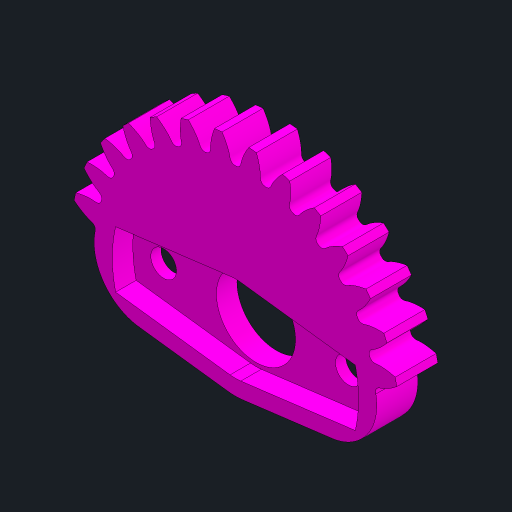
# Autodesk Inventor part: Servo Gear v3
Saved by Autodesk Inventor 2023.2 (Build 272271030, 271C)
## iProperties
Created: 2024-02-19
Part Number: Servo Gear v3
Material: Generic
Document SubType Name: Modeling
Designer: robpl
Density: 1 g/cm^3
Appearance: Magenta
Author: robpl
Autodesk Inventor part; units mm, degrees
ref_plane "YZ Plane" through (0, 0, 0) normal (1, 0, 0) x (0, 1, 0)
ref_plane "XZ Plane" through (0, 0, 0) normal (0, 1, 0) x (-1, 0, 0)
ref_plane "XY Plane" through (0, 0, 0) normal (0, 0, 1) x (1, 0, 0)
sketch "Sketch1" plane through (0, 0, 0) normal (0, 0, 1) x (1, 0, 0)
  spline S0 degree 3 poles (-1.3052, 15.9467) (-1.2453, 15.8516) (-1.1554, 15.709) (-1.0449, 15.5134) (-0.9655, 15.3647) (-0.8902, 15.2139) (-0.8193, 15.061) (-0.7533, 14.9059) (-0.6926, 14.7486) (-0.6381, 14.5891) (-0.5901, 14.4275) (-0.5589, 14.2906) (-0.5363, 14.1805) (-0.5125, 14.0995) (-0.4803, 14.0215) (-0.4383, 13.9482) (-0.3941, 13.8934) (-0.3542, 13.8537) (-0.3204, 13.8285) (-0.2858, 13.8043) (-0.2476, 13.7862) (-0.2089, 13.7695) (-0.1678, 13.7596) (-0.1265, 13.7512) (-0.0702, 13.7492) (0, 13.7505) (0.0702, 13.7492) (0.1265, 13.7512) (0.1678, 13.7596) (0.2089, 13.7695) (0.2476, 13.7862) (0.2858, 13.8043) (0.3204, 13.8285) (0.3542, 13.8537) (0.3941, 13.8934) (0.4383, 13.9482) (0.4803, 14.0215) (0.5125, 14.0995) (0.5363, 14.1805) (0.5589, 14.2906) (0.5901, 14.4275) (0.6381, 14.5891) (0.6926, 14.7486) (0.7533, 14.9059) (0.8193, 15.061) (0.8902, 15.2139) (0.9655, 15.3647) (1.0449, 15.5134) (1.1554, 15.709) (1.2453, 15.8516) (1.3052, 15.9467) knots 0 0 0 0 0.033702 0.050555 0.067407 0.084259 0.101111 0.117963 0.134815 0.151667 0.168518 0.185368 0.193792 0.202215 0.210638 0.219058 0.227476 0.231688 0.235901 0.240112 0.244326 0.248537 0.252749 0.256961 0.261174 0.2696 0.278026 0.282239 0.286451 0.290663 0.294874 0.299088 0.303299 0.307512 0.311724 0.320142 0.328562 0.336985 0.345408 0.353832 0.370682 0.387533 0.404385 0.421237 0.438089 0.454941 0.471793 0.488645 0.505498 0.5392 0.5392 0.5392 0.5392
  circle A0 centre (0, 0) radius 13.75 construction
  circle A1 centre (0, 0) radius 14.0954 construction
  circle A2 centre (0, 0) radius 15 construction
  circle A3 centre (0, 0) radius 16
  point P0 (-1.1285, 15.6597)
  point P1 (-1.0454, 15.513)
  point P2 (-0.9661, 15.3643)
  point P3 (-0.8909, 15.2135)
  point P4 (-0.8201, 15.0606)
  point P5 (-0.7542, 14.9055)
  point P6 (-0.6936, 14.7483)
  point P7 (-0.6392, 14.5888)
  point P8 (-0.5919, 14.4271)
  point P9 (-0.5535, 14.263)
  point P10 (-0.5352, 14.1808)
  point P11 (-0.5111, 14.1)
  point P12 (-0.4787, 14.0223)
  point P13 (-0.4365, 13.9494)
  point P14 (-0.3838, 13.8838)
  point P15 (-0.3535, 13.8545)
  point P16 (-0.3202, 13.8287)
  point P17 (-0.2852, 13.8053)
  point P18 (-0.2475, 13.7864)
  point P19 (-0.2085, 13.7706)
  point P20 (-0.1678, 13.7598)
  point P21 (-0.1263, 13.7524)
  point P22 (-0.0843, 13.75)
  point P23 (0, 13.75)
  point P24 (0.0843, 13.75)
  point P25 (0.1263, 13.7524)
  point P26 (0.1678, 13.7598)
  point P27 (0.2085, 13.7706)
  point P28 (0.2475, 13.7864)
  point P29 (0.2852, 13.8053)
  point P30 (0.3202, 13.8287)
  point P31 (0.3535, 13.8545)
  point P32 (0.3838, 13.8838)
  point P33 (0.4365, 13.9494)
  point P34 (0.4787, 14.0223)
  point P35 (0.5111, 14.1)
  point P36 (0.5352, 14.1808)
  point P37 (0.5535, 14.263)
  point P38 (0.5919, 14.4271)
  point P39 (0.6392, 14.5888)
  point P40 (0.6936, 14.7483)
  point P41 (0.7542, 14.9055)
  point P42 (0.8201, 15.0606)
  point P43 (0.8909, 15.2135)
  point P44 (0.9661, 15.3643)
  point P45 (1.0454, 15.513)
  point P46 (1.1285, 15.6597)
  constraints: 4 centre point, 2 point on circle, 103 other
extrude "Extrusion1" add sketch "Sketch1" against normal blind 4
extrude "Extrusion2" cut sketch "Sketch1" against normal through all contours A3 S0 picked at (-0.1198, 15.1654)
pattern_circular "Circular Pattern1" count 30 over 360 about axis through (0, 0, 0) along (0, 0, -1) of "Extrusion2"
sketch "Sketch2" plane through (0, 0, 0) normal (0, 0, 1) x (1, 0, 0)
  line L0 (-16, 0) -> (16, 0)
  arc A0 (-16.25, 1.9843) -> (-16.25, -1.9843) centre (-16, 0) ccw
  arc A1 (16.25, -1.9843) -> (16.25, 1.9843) centre (16, 0) ccw
  line L1 (0.5, 3.9686) -> (16.25, 1.9843)
  line L2 (16.25, -1.9843) -> (0.5, -3.9686)
  line L3 (-0.5, -3.9686) -> (-16.25, -1.9843)
  line L4 (-16.25, 1.9843) -> (-0.5, 3.9686)
  arc A2 (-0.5, -3.9686) -> (0.5, -3.9686) centre (0, 0) ccw
  arc A3 (0.5, 3.9686) -> (-0.5, 3.9686) centre (0, 0) ccw
  line L5 (16.275, 2.1827) -> (0.525, 4.1671)
  arc A4 (0.525, 4.1671) -> (-0.525, 4.1671) centre (0, 0) ccw
  line L6 (-0.525, 4.1671) -> (-16.275, 2.1827)
  arc A5 (-16.275, 2.1827) -> (-16.275, -2.1827) centre (-16, 0) ccw
  line L7 (-16.275, -2.1827) -> (-0.525, -4.1671)
  arc A6 (-0.525, -4.1671) -> (0.525, -4.1671) centre (0, 0) ccw
  line L8 (0.525, -4.1671) -> (16.275, -2.1827)
  arc A7 (16.275, -2.1827) -> (16.275, 2.1827) centre (16, 0) ccw
  circle A8 centre (0, 0) radius 12
  point P0 (11.6778, 2.7619)
  point P1 (-11.6778, 2.7619)
  point P2 (-11.6778, -2.7619)
  point P3 (11.6778, -2.7619)
  dimension "d8" = 32
  dimension "d9" = 4
  dimension "d10" = 4
  dimension "d11" = 4
  dimension "d12" = 0.2
  dimension "d13" = 24
  constraints: 18 end point, 16 point on circle, 9 centre point, 5 coincident, 5 tangent, 4 parallel, 1 horizontal, 1 midpoint, 7 other
  measures "d8" distance of L0.start L0.end
  measures "d9" diameter of A0
  measures "d10" diameter of A1
  measures "d11" radius of A2
  measures "d12" distance between parallel lines of L1 L5
  measures "d13" diameter of A8
extrude "Extrusion3" cut sketch "Sketch2" against normal blind 2 contours A8 L4 A3 L1 L0 | L0 A8 L2 A2 L3 | A8 L6 A4 L5 L1 A3 L4 | L3 A2 L2 A8 L8 A6 L7
sketch "Sketch3" plane through (0, 0, -2) normal (0, 0, 1) x (1, 0, 0)
  circle A0 centre (0, 0) radius 4.2
  line L0 (0.525, 4.1671) -> (11.6778, 2.7619) projected
  circle A1 centre (0, 0) radius 3.85
  dimension "d31" = 7.7
  constraints: 2 coincident, 1 centre point, 3 other
  measures "d31" diameter of A1
extrude "Extrusion4" cut sketch "Sketch3" against normal through all contours A1
sketch "Sketch4" plane through (0, 0, -4) normal (0, 0, -1) x (-1, 0, 0)
  point P0 (0, 0)
  point P1 (-9, 0)
  point P2 (9, 0)
  dimension "d18" = 18
  dimension "d19" = 9
  constraints: 2 horizontal alignment
  measures "d18" distance of point (-9, 0) point (9, 0)
  measures "d19" distance of point (0, 0) point (-9, 0)
hole "Hole1" at (9, 0, -4) at (-9, 0, -4) direction (0, 0, 1) diameter 2.5 end through all counterbore diameter 6 counterbore depth 1
sketch "Sketch6" plane through (0, 0, 0) normal (0, 0, 1) x (1, 0, 0)
  arc A0 (0.525, 4.1671) -> (-0.525, 4.1671) centre (0, 0) ccw projected
  line L0 (0.525, 4.1671) -> (11.6778, 2.7619) projected
  arc A1 (11.6778, -2.7619) -> (11.6778, 2.7619) centre (0, 0) ccw projected
  line L1 (11.6778, -2.7619) -> (0.525, -4.1671) projected
  line L2 (-0.525, -4.1671) -> (-11.6778, -2.7619) projected
  arc A2 (-11.6778, 2.7619) -> (-11.6778, -2.7619) centre (0, 0) ccw projected
  line L3 (-11.6778, 2.7619) -> (-0.525, 4.1671) projected
  arc A3 (-4.5922, 15.3268) -> (-5.2937, 15.0989) centre (0, 0) ccw projected
  arc A4 (-7.6784, 14.0371) -> (-8.3173, 13.6683) centre (0, 0) ccw projected
  arc A5 (-10.4291, 12.134) -> (-10.9773, 11.6404) centre (0, 0) ccw projected
  arc A6 (-12.724, 9.7005) -> (-13.1576, 9.1037) centre (0, 0) ccw projected
  arc A7 (-14.4628, 6.843) -> (-14.7629, 6.1691) centre (0, 0) ccw projected
  arc A8 (-15.5695, 3.6865) -> (-15.7229, 2.9649) centre (0, 0) ccw projected
  spline S0 degree 3 poles (-15.7229, 2.9649) (-15.6346, 2.8954) (-15.5022, 2.7911) (-15.3192, 2.6607) (-15.1796, 2.5662) (-15.0375, 2.4756) (-14.8928, 2.3892) (-14.7455, 2.3073) (-14.5954, 2.2305) (-14.4425, 2.1596) (-14.2868, 2.095) (-14.1538, 2.0496) (-14.0467, 2.0157) (-13.9687, 1.9835) (-13.8945, 1.9433) (-13.8259, 1.8939) (-13.7761, 1.8442) (-13.7408, 1.8003) (-13.7193, 1.7641) (-13.6988, 1.7271) (-13.6848, 1.6873) (-13.6722, 1.647) (-13.6667, 1.6052) (-13.6627, 1.5632) (-13.6666, 1.507) (-13.6752, 1.4373) (-13.6812, 1.3674) (-13.6891, 1.3116) (-13.7017, 1.2714) (-13.7159, 1.2316) (-13.7366, 1.1948) (-13.7586, 1.1587) (-13.7862, 1.1269) (-13.8149, 1.0959) (-13.8584, 1.0603) (-13.9176, 1.022) (-13.9949, 0.988) (-14.0759, 0.9641) (-14.1589, 0.9489) (-14.2707, 0.9379) (-14.4102, 0.9212) (-14.5759, 0.8904) (-14.7402, 0.8528) (-14.903, 0.8089) (-15.0641, 0.7594) (-15.2236, 0.705) (-15.3815, 0.6459) (-15.5376, 0.5825) (-15.7438, 0.493) (-15.895, 0.4185) (-15.9957, 0.3688) knots 0 0 0 0 0.062504 0.093759 0.125013 0.156267 0.187521 0.218774 0.250028 0.281281 0.312533 0.343783 0.359406 0.375028 0.39065 0.406265 0.421876 0.429689 0.437502 0.445312 0.453126 0.460936 0.468749 0.47656 0.484373 0.5 0.515627 0.52344 0.531251 0.539064 0.546874 0.554688 0.562498 0.570311 0.578124 0.593735 0.60935 0.624972 0.640594 0.656217 0.687467 0.718719 0.749972 0.781226 0.812479 0.843733 0.874987 0.906241 0.937496 1 1 1 1 projected
  arc A9 (-15.9957, 0.3688) -> (-15.9957, -0.3688) centre (0, 0) ccw projected
  spline S1 degree 3 poles (-15.9957, -0.3688) (-15.895, -0.4185) (-15.7438, -0.493) (-15.5376, -0.5825) (-15.3815, -0.6459) (-15.2236, -0.705) (-15.0641, -0.7594) (-14.903, -0.8089) (-14.7402, -0.8528) (-14.5759, -0.8904) (-14.4102, -0.9212) (-14.2707, -0.9379) (-14.1589, -0.9489) (-14.0759, -0.9641) (-13.9949, -0.988) (-13.9176, -1.022) (-13.8584, -1.0603) (-13.8149, -1.0959) (-13.7862, -1.1269) (-13.7586, -1.1587) (-13.7366, -1.1948) (-13.7159, -1.2316) (-13.7017, -1.2714) (-13.6891, -1.3116) (-13.6812, -1.3674) (-13.6752, -1.4373) (-13.6666, -1.507) (-13.6627, -1.5632) (-13.6667, -1.6052) (-13.6722, -1.647) (-13.6848, -1.6873) (-13.6988, -1.7271) (-13.7193, -1.7641) (-13.7408, -1.8003) (-13.7761, -1.8442) (-13.8259, -1.8939) (-13.8945, -1.9433) (-13.9687, -1.9835) (-14.0467, -2.0157) (-14.1538, -2.0496) (-14.2868, -2.095) (-14.4425, -2.1596) (-14.5954, -2.2305) (-14.7455, -2.3073) (-14.8928, -2.3892) (-15.0375, -2.4756) (-15.1796, -2.5662) (-15.3192, -2.6607) (-15.5022, -2.7911) (-15.6346, -2.8954) (-15.7229, -2.9649) knots 0 0 0 0 0.062504 0.093759 0.125013 0.156267 0.187521 0.218774 0.250028 0.281281 0.312533 0.343783 0.359406 0.375028 0.39065 0.406265 0.421876 0.429689 0.437502 0.445312 0.453126 0.460936 0.468749 0.47656 0.484373 0.5 0.515627 0.52344 0.531251 0.539064 0.546874 0.554688 0.562498 0.570311 0.578124 0.593735 0.60935 0.624972 0.640594 0.656217 0.687467 0.718719 0.749972 0.781226 0.812479 0.843733 0.874987 0.906241 0.937496 1 1 1 1 projected
  arc A10 (-15.7229, -2.9649) -> (-15.5695, -3.6865) centre (0, 0) ccw projected
  spline S2 degree 3 poles (-15.5695, -3.6865) (-15.4606, -3.7141) (-15.2972, -3.7555) (-15.077, -3.8002) (-14.911, -3.8298) (-14.7444, -3.8547) (-14.577, -3.8749) (-14.4091, -3.8897) (-14.2408, -3.8989) (-14.0723, -3.9014) (-13.9037, -3.8971) (-13.7638, -3.8845) (-13.6522, -3.8719) (-13.5678, -3.8696) (-13.4837, -3.8761) (-13.401, -3.8933) (-13.3352, -3.9185) (-13.2851, -3.9442) (-13.2507, -3.9685) (-13.217, -3.994) (-13.188, -4.0247) (-13.1601, -4.0564) (-13.138, -4.0923) (-13.1173, -4.1291) (-13.098, -4.182) (-13.0775, -4.2491) (-13.0546, -4.3155) (-13.0391, -4.3696) (-13.0343, -4.4116) (-13.031, -4.4537) (-13.035, -4.4957) (-13.0404, -4.5375) (-13.0527, -4.5779) (-13.0662, -4.6179) (-13.0916, -4.6681) (-13.13, -4.7271) (-13.1869, -4.7897) (-13.2511, -4.8444) (-13.3207, -4.8921) (-13.4184, -4.9476) (-13.539, -5.0196) (-13.6779, -5.1152) (-13.8128, -5.2163) (-13.9435, -5.3226) (-14.0706, -5.4333) (-14.1942, -5.548) (-14.3144, -5.6662) (-14.4312, -5.7876) (-14.5832, -5.9532) (-14.691, -6.0827) (-14.7629, -6.1691) knots 0 0 0 0 0.062504 0.093759 0.125013 0.156267 0.187521 0.218774 0.250028 0.281281 0.312533 0.343783 0.359406 0.375028 0.39065 0.406265 0.421876 0.429689 0.437502 0.445312 0.453126 0.460936 0.468749 0.47656 0.484373 0.5 0.515627 0.52344 0.531251 0.539064 0.546874 0.554688 0.562498 0.570311 0.578124 0.593735 0.60935 0.624972 0.640594 0.656217 0.687467 0.718719 0.749972 0.781226 0.812479 0.843733 0.874987 0.906241 0.937496 1 1 1 1 projected
  arc A11 (-14.7629, -6.1691) -> (-14.4628, -6.843) centre (0, 0) ccw projected
  spline S3 degree 3 poles (-14.4628, -6.843) (-14.3505, -6.8474) (-14.1821, -6.8539) (-13.9574, -6.8518) (-13.789, -6.8462) (-13.6207, -6.836) (-13.4528, -6.8209) (-13.2855, -6.8005) (-13.119, -6.7745) (-12.9536, -6.742) (-12.7897, -6.7027) (-12.6554, -6.6613) (-12.5488, -6.6258) (-12.4668, -6.6059) (-12.3832, -6.5948) (-12.2987, -6.5945) (-12.2291, -6.6054) (-12.1748, -6.6202) (-12.136, -6.6368) (-12.0978, -6.6547) (-12.063, -6.6787) (-12.0292, -6.7039) (-12.0001, -6.7344) (-11.9721, -6.7661) (-11.9423, -6.8138) (-11.9083, -6.8753) (-11.8721, -6.9354) (-11.8457, -6.9851) (-11.8322, -7.0251) (-11.8203, -7.0656) (-11.8154, -7.1076) (-11.812, -7.1496) (-11.8156, -7.1917) (-11.8206, -7.2336) (-11.8349, -7.288) (-11.8603, -7.3537) (-11.9029, -7.4267) (-11.9543, -7.4936) (-12.0125, -7.5547) (-12.0965, -7.6293) (-12.1995, -7.7248) (-12.3155, -7.8472) (-12.4264, -7.9741) (-12.5322, -8.1053) (-12.6335, -8.2401) (-12.7305, -8.3779) (-12.8235, -8.5185) (-12.9125, -8.6616) (-13.0267, -8.8551) (-13.1053, -9.0042) (-13.1576, -9.1037) knots 0 0 0 0 0.062504 0.093759 0.125013 0.156267 0.187521 0.218774 0.250028 0.281281 0.312533 0.343783 0.359406 0.375028 0.39065 0.406265 0.421876 0.429689 0.437502 0.445312 0.453126 0.460936 0.468749 0.47656 0.484373 0.5 0.515627 0.52344 0.531251 0.539064 0.546874 0.554688 0.562498 0.570311 0.578124 0.593735 0.60935 0.624972 0.640594 0.656217 0.687467 0.718719 0.749972 0.781226 0.812479 0.843733 0.874987 0.906241 0.937496 1 1 1 1 projected
  arc A12 (-13.1576, -9.1037) -> (-12.724, -9.7005) centre (0, 0) ccw projected
  spline S4 degree 3 poles (-12.724, -9.7005) (-12.6133, -9.6814) (-12.4472, -9.6528) (-12.2278, -9.604) (-12.0642, -9.5635) (-11.9018, -9.5185) (-11.7407, -9.4689) (-11.5813, -9.4142) (-11.4238, -9.354) (-11.2688, -9.2878) (-11.1166, -9.2153) (-10.9939, -9.1469) (-10.897, -9.09) (-10.8209, -9.0536) (-10.7414, -9.0253) (-10.6588, -9.0074) (-10.5885, -9.0036) (-10.5323, -9.0068) (-10.491, -9.015) (-10.4498, -9.0245) (-10.4109, -9.0408) (-10.3725, -9.0584) (-10.3377, -9.0822) (-10.3038, -9.1074) (-10.2646, -9.1479) (-10.2186, -9.2009) (-10.1707, -9.2522) (-10.1345, -9.2953) (-10.1131, -9.3317) (-10.093, -9.3688) (-10.0795, -9.4088) (-10.0674, -9.4493) (-10.0622, -9.4912) (-10.0584, -9.5332) (-10.0611, -9.5894) (-10.0722, -9.6589) (-10.0986, -9.7392) (-10.1351, -9.8153) (-10.1793, -9.8872) (-10.246, -9.9776) (-10.3269, -10.0924) (-10.4149, -10.2362) (-10.4969, -10.3835) (-10.5732, -10.5338) (-10.6442, -10.6866) (-10.7105, -10.8416) (-10.7722, -10.9985) (-10.8295, -11.1569) (-10.901, -11.37) (-10.9468, -11.5322) (-10.9773, -11.6404) knots 0 0 0 0 0.062504 0.093759 0.125013 0.156267 0.187521 0.218774 0.250028 0.281281 0.312533 0.343783 0.359406 0.375028 0.39065 0.406265 0.421876 0.429689 0.437502 0.445312 0.453126 0.460936 0.468749 0.47656 0.484373 0.5 0.515627 0.52344 0.531251 0.539064 0.546874 0.554688 0.562498 0.570311 0.578124 0.593735 0.60935 0.624972 0.640594 0.656217 0.687467 0.718719 0.749972 0.781226 0.812479 0.843733 0.874987 0.906241 0.937496 1 1 1 1 projected
  arc A13 (-10.9773, -11.6404) -> (-10.4291, -12.134) centre (0, 0) ccw projected
  spline S5 degree 3 poles (-10.4291, -12.134) (-10.3248, -12.0923) (-10.1683, -12.0298) (-9.9638, -11.9364) (-9.8122, -11.8628) (-9.6627, -11.785) (-9.5155, -11.703) (-9.3709, -11.6163) (-9.2294, -11.5248) (-9.0915, -11.4278) (-8.9577, -11.3252) (-8.8519, -11.2328) (-8.769, -11.157) (-8.7021, -11.1055) (-8.6302, -11.0613) (-8.5532, -11.0267) (-8.4852, -11.0083) (-8.4295, -10.9997) (-8.3874, -10.9992) (-8.3452, -10.9999) (-8.3037, -11.0077) (-8.2625, -11.017) (-8.2235, -11.0331) (-8.1851, -11.0506) (-8.1384, -11.0821) (-8.0824, -11.1244) (-8.0248, -11.1646) (-7.9805, -11.1993) (-7.9519, -11.2304) (-7.9245, -11.2625) (-7.903, -11.2988) (-7.8828, -11.3359) (-7.869, -11.3758) (-7.8565, -11.4161) (-7.8475, -11.4716) (-7.8439, -11.542) (-7.8531, -11.626) (-7.8729, -11.708) (-7.9012, -11.7875) (-7.9476, -11.8898) (-8.0029, -12.019) (-8.0591, -12.1779) (-8.1087, -12.339) (-8.152, -12.5019) (-8.1897, -12.6662) (-8.2223, -12.8315) (-8.2501, -12.9978) (-8.2732, -13.1647) (-8.2988, -13.388) (-8.3099, -13.5562) (-8.3173, -13.6683) knots 0 0 0 0 0.062504 0.093759 0.125013 0.156267 0.187521 0.218774 0.250028 0.281281 0.312533 0.343783 0.359406 0.375028 0.39065 0.406265 0.421876 0.429689 0.437502 0.445312 0.453126 0.460936 0.468749 0.47656 0.484373 0.5 0.515627 0.52344 0.531251 0.539064 0.546874 0.554688 0.562498 0.570311 0.578124 0.593735 0.60935 0.624972 0.640594 0.656217 0.687467 0.718719 0.749972 0.781226 0.812479 0.843733 0.874987 0.906241 0.937496 1 1 1 1 projected
  arc A14 (-8.3173, -13.6683) -> (-7.6784, -14.0371) centre (0, 0) ccw projected
  spline S6 degree 3 poles (-7.6784, -14.0371) (-7.585, -13.9747) (-7.4449, -13.881) (-7.2644, -13.7472) (-7.1314, -13.6437) (-7.0013, -13.5365) (-6.8744, -13.4256) (-6.751, -13.3108) (-6.6315, -13.1918) (-6.5169, -13.0683) (-6.4073, -12.9402) (-6.3231, -12.8277) (-6.2577, -12.7364) (-6.203, -12.6721) (-6.1419, -12.614) (-6.0737, -12.564) (-6.011, -12.5319) (-5.9584, -12.512) (-5.9172, -12.5027) (-5.8758, -12.4946) (-5.8336, -12.4936) (-5.7914, -12.4941) (-5.7498, -12.5017) (-5.7087, -12.5109) (-5.6564, -12.532) (-5.5928, -12.5617) (-5.5282, -12.5891) (-5.4776, -12.6138) (-5.4432, -12.6383) (-5.4097, -12.664) (-5.3811, -12.6951) (-5.3537, -12.7271) (-5.3319, -12.7633) (-5.3113, -12.8001) (-5.2909, -12.8525) (-5.2728, -12.9206) (-5.2643, -13.0047) (-5.2666, -13.089) (-5.2777, -13.1727) (-5.3019, -13.2824) (-5.3291, -13.4202) (-5.351, -13.5874) (-5.3661, -13.7553) (-5.3746, -13.9236) (-5.3773, -14.0921) (-5.3748, -14.2607) (-5.3674, -14.429) (-5.3553, -14.5971) (-5.334, -14.8209) (-5.3098, -14.9877) (-5.2937, -15.0989) knots 0 0 0 0 0.062504 0.093759 0.125013 0.156267 0.187521 0.218774 0.250028 0.281281 0.312533 0.343783 0.359406 0.375028 0.39065 0.406265 0.421876 0.429689 0.437502 0.445312 0.453126 0.460936 0.468749 0.47656 0.484373 0.5 0.515627 0.52344 0.531251 0.539064 0.546874 0.554688 0.562498 0.570311 0.578124 0.593735 0.60935 0.624972 0.640594 0.656217 0.687467 0.718719 0.749972 0.781226 0.812479 0.843733 0.874987 0.906241 0.937496 1 1 1 1 projected
  arc A15 (-5.2937, -15.0989) -> (-4.5922, -15.3268) centre (0, 0) ccw projected
  spline S7 degree 3 poles (-4.5922, -15.3268) (-4.5138, -15.2463) (-4.3962, -15.1255) (-4.2474, -14.9571) (-4.1389, -14.8282) (-4.0339, -14.6963) (-3.9328, -14.5615) (-3.836, -14.4235) (-3.7439, -14.2823) (-3.6574, -14.1377) (-3.5769, -13.9895) (-3.5179, -13.8621) (-3.4729, -13.7591) (-3.4328, -13.6849) (-3.3851, -13.6153) (-3.3288, -13.5522) (-3.2741, -13.5078) (-3.2268, -13.4774) (-3.1885, -13.4597) (-3.1496, -13.4432) (-3.1085, -13.4335) (-3.0671, -13.4252) (-3.0249, -13.424) (-2.9827, -13.4244) (-2.9273, -13.4342) (-2.8589, -13.45) (-2.79, -13.4634) (-2.7353, -13.477) (-2.6966, -13.4938) (-2.6585, -13.512) (-2.6241, -13.5365) (-2.5906, -13.5621) (-2.5617, -13.5929) (-2.5339, -13.6246) (-2.5031, -13.6717) (-2.4712, -13.7345) (-2.4454, -13.815) (-2.4301, -13.898) (-2.4237, -13.9821) (-2.4245, -14.0945) (-2.4224, -14.2349) (-2.4091, -14.403) (-2.3889, -14.5703) (-2.3622, -14.7368) (-2.3299, -14.9022) (-2.2924, -15.0665) (-2.2501, -15.2297) (-2.2034, -15.3916) (-2.136, -15.606) (-2.0777, -15.7641) (-2.0388, -15.8696) knots 0 0 0 0 0.062504 0.093759 0.125013 0.156267 0.187521 0.218774 0.250028 0.281281 0.312533 0.343783 0.359406 0.375028 0.39065 0.406265 0.421876 0.429689 0.437502 0.445312 0.453126 0.460936 0.468749 0.47656 0.484373 0.5 0.515627 0.52344 0.531251 0.539064 0.546874 0.554688 0.562498 0.570311 0.578124 0.593735 0.60935 0.624972 0.640594 0.656217 0.687467 0.718719 0.749972 0.781226 0.812479 0.843733 0.874987 0.906241 0.937496 1 1 1 1 projected
  arc A16 (-2.0388, -15.8696) -> (-1.3052, -15.9467) centre (0, 0) ccw projected
  spline S8 degree 3 poles (-1.3052, -15.9467) (-1.2453, -15.8516) (-1.1554, -15.709) (-1.0449, -15.5134) (-0.9655, -15.3647) (-0.8902, -15.2139) (-0.8193, -15.061) (-0.7533, -14.9059) (-0.6926, -14.7486) (-0.6381, -14.5891) (-0.5901, -14.4275) (-0.5589, -14.2906) (-0.5363, -14.1805) (-0.5125, -14.0995) (-0.4803, -14.0215) (-0.4383, -13.9482) (-0.3941, -13.8934) (-0.3542, -13.8537) (-0.3204, -13.8285) (-0.2858, -13.8043) (-0.2476, -13.7862) (-0.2089, -13.7695) (-0.1678, -13.7596) (-0.1265, -13.7512) (-0.0702, -13.7492) (0, -13.7505) (0.0702, -13.7492) (0.1265, -13.7512) (0.1678, -13.7596) (0.2089, -13.7695) (0.2476, -13.7862) (0.2858, -13.8043) (0.3204, -13.8285) (0.3542, -13.8537) (0.3941, -13.8934) (0.4383, -13.9482) (0.4803, -14.0215) (0.5125, -14.0995) (0.5363, -14.1805) (0.5589, -14.2906) (0.5901, -14.4275) (0.6381, -14.5891) (0.6926, -14.7486) (0.7533, -14.9059) (0.8193, -15.061) (0.8902, -15.2139) (0.9655, -15.3647) (1.0449, -15.5134) (1.1554, -15.709) (1.2453, -15.8516) (1.3052, -15.9467) knots 0 0 0 0 0.062504 0.093759 0.125013 0.156267 0.187521 0.218774 0.250028 0.281281 0.312533 0.343783 0.359406 0.375028 0.39065 0.406265 0.421876 0.429689 0.437502 0.445312 0.453126 0.460936 0.468749 0.47656 0.484373 0.5 0.515627 0.52344 0.531251 0.539064 0.546874 0.554688 0.562498 0.570311 0.578124 0.593735 0.60935 0.624972 0.640594 0.656217 0.687467 0.718719 0.749972 0.781226 0.812479 0.843733 0.874987 0.906241 0.937496 1 1 1 1 projected
  arc A17 (1.3052, -15.9467) -> (2.0388, -15.8696) centre (0, 0) ccw projected
  spline S9 degree 3 poles (2.0388, -15.8696) (2.0777, -15.7641) (2.136, -15.606) (2.2034, -15.3916) (2.2501, -15.2297) (2.2924, -15.0665) (2.3299, -14.9022) (2.3622, -14.7368) (2.3889, -14.5703) (2.4091, -14.403) (2.4224, -14.2349) (2.4245, -14.0945) (2.4237, -13.9821) (2.4301, -13.898) (2.4454, -13.815) (2.4712, -13.7345) (2.5031, -13.6717) (2.5339, -13.6246) (2.5617, -13.5929) (2.5906, -13.5621) (2.6241, -13.5365) (2.6585, -13.512) (2.6966, -13.4938) (2.7353, -13.477) (2.79, -13.4634) (2.8589, -13.45) (2.9273, -13.4342) (2.9827, -13.4244) (3.0249, -13.424) (3.0671, -13.4252) (3.1085, -13.4335) (3.1496, -13.4432) (3.1885, -13.4597) (3.2268, -13.4774) (3.2741, -13.5078) (3.3288, -13.5522) (3.3851, -13.6153) (3.4328, -13.6849) (3.4729, -13.7591) (3.5179, -13.8621) (3.5769, -13.9895) (3.6574, -14.1377) (3.7439, -14.2823) (3.836, -14.4235) (3.9328, -14.5615) (4.0339, -14.6963) (4.1389, -14.8282) (4.2474, -14.9571) (4.3962, -15.1255) (4.5138, -15.2463) (4.5922, -15.3268) knots 0 0 0 0 0.062504 0.093759 0.125013 0.156267 0.187521 0.218774 0.250028 0.281281 0.312533 0.343783 0.359406 0.375028 0.39065 0.406265 0.421876 0.429689 0.437502 0.445312 0.453126 0.460936 0.468749 0.47656 0.484373 0.5 0.515627 0.52344 0.531251 0.539064 0.546874 0.554688 0.562498 0.570311 0.578124 0.593735 0.60935 0.624972 0.640594 0.656217 0.687467 0.718719 0.749972 0.781226 0.812479 0.843733 0.874987 0.906241 0.937496 1 1 1 1 projected
  arc A18 (4.5922, -15.3268) -> (5.2937, -15.0989) centre (0, 0) ccw projected
  spline S10 degree 3 poles (5.2937, -15.0989) (5.3098, -14.9877) (5.334, -14.8209) (5.3553, -14.5971) (5.3674, -14.429) (5.3748, -14.2607) (5.3773, -14.0921) (5.3746, -13.9236) (5.3661, -13.7553) (5.351, -13.5874) (5.3291, -13.4202) (5.3019, -13.2824) (5.2777, -13.1727) (5.2666, -13.089) (5.2643, -13.0047) (5.2728, -12.9206) (5.2909, -12.8525) (5.3113, -12.8001) (5.3319, -12.7633) (5.3537, -12.7271) (5.3811, -12.6951) (5.4097, -12.664) (5.4432, -12.6383) (5.4776, -12.6138) (5.5282, -12.5891) (5.5928, -12.5617) (5.6564, -12.532) (5.7087, -12.5109) (5.7498, -12.5017) (5.7914, -12.4941) (5.8336, -12.4936) (5.8758, -12.4946) (5.9172, -12.5027) (5.9584, -12.512) (6.011, -12.5319) (6.0737, -12.564) (6.1419, -12.614) (6.203, -12.6721) (6.2577, -12.7364) (6.3231, -12.8277) (6.4073, -12.9402) (6.5169, -13.0683) (6.6315, -13.1918) (6.751, -13.3108) (6.8744, -13.4256) (7.0013, -13.5365) (7.1314, -13.6437) (7.2644, -13.7472) (7.4449, -13.881) (7.585, -13.9747) (7.6784, -14.0371) knots 0 0 0 0 0.062504 0.093759 0.125013 0.156267 0.187521 0.218774 0.250028 0.281281 0.312533 0.343783 0.359406 0.375028 0.39065 0.406265 0.421876 0.429689 0.437502 0.445312 0.453126 0.460936 0.468749 0.47656 0.484373 0.5 0.515627 0.52344 0.531251 0.539064 0.546874 0.554688 0.562498 0.570311 0.578124 0.593735 0.60935 0.624972 0.640594 0.656217 0.687467 0.718719 0.749972 0.781226 0.812479 0.843733 0.874987 0.906241 0.937496 1 1 1 1 projected
  arc A19 (7.6784, -14.0371) -> (8.3173, -13.6683) centre (0, 0) ccw projected
  spline S11 degree 3 poles (8.3173, -13.6683) (8.3099, -13.5562) (8.2988, -13.388) (8.2732, -13.1647) (8.2501, -12.9978) (8.2223, -12.8315) (8.1897, -12.6662) (8.152, -12.5019) (8.1087, -12.339) (8.0591, -12.1779) (8.0029, -12.019) (7.9476, -11.8898) (7.9012, -11.7875) (7.8729, -11.708) (7.8531, -11.626) (7.8439, -11.542) (7.8475, -11.4716) (7.8565, -11.4161) (7.869, -11.3758) (7.8828, -11.3359) (7.903, -11.2988) (7.9245, -11.2625) (7.9519, -11.2304) (7.9805, -11.1993) (8.0248, -11.1646) (8.0824, -11.1244) (8.1384, -11.0821) (8.1851, -11.0506) (8.2235, -11.0331) (8.2625, -11.017) (8.3037, -11.0077) (8.3452, -10.9999) (8.3874, -10.9992) (8.4295, -10.9997) (8.4852, -11.0083) (8.5532, -11.0267) (8.6302, -11.0613) (8.7021, -11.1055) (8.769, -11.157) (8.8519, -11.2328) (8.9577, -11.3252) (9.0915, -11.4278) (9.2294, -11.5248) (9.3709, -11.6163) (9.5155, -11.703) (9.6627, -11.785) (9.8122, -11.8628) (9.9638, -11.9364) (10.1683, -12.0298) (10.3248, -12.0923) (10.4291, -12.134) knots 0 0 0 0 0.062504 0.093759 0.125013 0.156267 0.187521 0.218774 0.250028 0.281281 0.312533 0.343783 0.359406 0.375028 0.39065 0.406265 0.421876 0.429689 0.437502 0.445312 0.453126 0.460936 0.468749 0.47656 0.484373 0.5 0.515627 0.52344 0.531251 0.539064 0.546874 0.554688 0.562498 0.570311 0.578124 0.593735 0.60935 0.624972 0.640594 0.656217 0.687467 0.718719 0.749972 0.781226 0.812479 0.843733 0.874987 0.906241 0.937496 1 1 1 1 projected
  arc A20 (10.4291, -12.134) -> (10.9773, -11.6404) centre (0, 0) ccw projected
  spline S12 degree 3 poles (10.9773, -11.6404) (10.9468, -11.5322) (10.901, -11.37) (10.8295, -11.1569) (10.7722, -10.9985) (10.7105, -10.8416) (10.6442, -10.6866) (10.5732, -10.5338) (10.4969, -10.3835) (10.4149, -10.2362) (10.3269, -10.0924) (10.246, -9.9776) (10.1793, -9.8872) (10.1351, -9.8153) (10.0986, -9.7392) (10.0722, -9.6589) (10.0611, -9.5894) (10.0584, -9.5332) (10.0622, -9.4912) (10.0674, -9.4493) (10.0795, -9.4088) (10.093, -9.3688) (10.1131, -9.3317) (10.1345, -9.2953) (10.1707, -9.2522) (10.2186, -9.2009) (10.2646, -9.1479) (10.3038, -9.1074) (10.3377, -9.0822) (10.3725, -9.0584) (10.4109, -9.0408) (10.4498, -9.0245) (10.491, -9.015) (10.5323, -9.0068) (10.5885, -9.0036) (10.6588, -9.0074) (10.7414, -9.0253) (10.8209, -9.0536) (10.897, -9.09) (10.9939, -9.1469) (11.1166, -9.2153) (11.2688, -9.2878) (11.4238, -9.354) (11.5813, -9.4142) (11.7407, -9.4689) (11.9018, -9.5185) (12.0642, -9.5635) (12.2278, -9.604) (12.4472, -9.6528) (12.6133, -9.6814) (12.724, -9.7005) knots 0 0 0 0 0.062504 0.093759 0.125013 0.156267 0.187521 0.218774 0.250028 0.281281 0.312533 0.343783 0.359406 0.375028 0.39065 0.406265 0.421876 0.429689 0.437502 0.445312 0.453126 0.460936 0.468749 0.47656 0.484373 0.5 0.515627 0.52344 0.531251 0.539064 0.546874 0.554688 0.562498 0.570311 0.578124 0.593735 0.60935 0.624972 0.640594 0.656217 0.687467 0.718719 0.749972 0.781226 0.812479 0.843733 0.874987 0.906241 0.937496 1 1 1 1 projected
  arc A21 (12.724, -9.7005) -> (13.1576, -9.1037) centre (0, 0) ccw projected
  spline S13 degree 3 poles (13.1576, -9.1037) (13.1053, -9.0042) (13.0267, -8.8551) (12.9125, -8.6616) (12.8235, -8.5185) (12.7305, -8.3779) (12.6335, -8.2401) (12.5322, -8.1053) (12.4264, -7.9741) (12.3155, -7.8472) (12.1995, -7.7248) (12.0965, -7.6293) (12.0125, -7.5547) (11.9543, -7.4936) (11.9029, -7.4267) (11.8603, -7.3537) (11.8349, -7.288) (11.8206, -7.2336) (11.8156, -7.1917) (11.812, -7.1496) (11.8154, -7.1076) (11.8203, -7.0656) (11.8322, -7.0251) (11.8457, -6.9851) (11.8721, -6.9354) (11.9083, -6.8753) (11.9423, -6.8138) (11.9721, -6.7661) (12.0001, -6.7344) (12.0292, -6.7039) (12.063, -6.6787) (12.0978, -6.6547) (12.136, -6.6368) (12.1748, -6.6202) (12.2291, -6.6054) (12.2987, -6.5945) (12.3832, -6.5948) (12.4668, -6.6059) (12.5488, -6.6258) (12.6554, -6.6613) (12.7897, -6.7027) (12.9536, -6.742) (13.119, -6.7745) (13.2855, -6.8005) (13.4528, -6.8209) (13.6207, -6.836) (13.789, -6.8462) (13.9574, -6.8518) (14.1821, -6.8539) (14.3505, -6.8474) (14.4628, -6.843) knots 0 0 0 0 0.062504 0.093759 0.125013 0.156267 0.187521 0.218774 0.250028 0.281281 0.312533 0.343783 0.359406 0.375028 0.39065 0.406265 0.421876 0.429689 0.437502 0.445312 0.453126 0.460936 0.468749 0.47656 0.484373 0.5 0.515627 0.52344 0.531251 0.539064 0.546874 0.554688 0.562498 0.570311 0.578124 0.593735 0.60935 0.624972 0.640594 0.656217 0.687467 0.718719 0.749972 0.781226 0.812479 0.843733 0.874987 0.906241 0.937496 1 1 1 1 projected
  arc A22 (14.4628, -6.843) -> (14.7629, -6.1691) centre (0, 0) ccw projected
  spline S14 degree 3 poles (14.7629, -6.1691) (14.691, -6.0827) (14.5832, -5.9532) (14.4312, -5.7876) (14.3144, -5.6662) (14.1942, -5.548) (14.0706, -5.4333) (13.9435, -5.3226) (13.8128, -5.2163) (13.6779, -5.1152) (13.539, -5.0196) (13.4184, -4.9476) (13.3207, -4.8921) (13.2511, -4.8444) (13.1869, -4.7897) (13.13, -4.7271) (13.0916, -4.6681) (13.0662, -4.6179) (13.0527, -4.5779) (13.0404, -4.5375) (13.035, -4.4957) (13.031, -4.4537) (13.0343, -4.4116) (13.0391, -4.3696) (13.0546, -4.3155) (13.0775, -4.2491) (13.098, -4.182) (13.1173, -4.1291) (13.138, -4.0923) (13.1601, -4.0564) (13.188, -4.0247) (13.217, -3.994) (13.2507, -3.9685) (13.2851, -3.9442) (13.3352, -3.9185) (13.401, -3.8933) (13.4837, -3.8761) (13.5678, -3.8696) (13.6522, -3.8719) (13.7638, -3.8845) (13.9037, -3.8971) (14.0723, -3.9014) (14.2408, -3.8989) (14.4091, -3.8897) (14.577, -3.8749) (14.7444, -3.8547) (14.911, -3.8298) (15.077, -3.8002) (15.2972, -3.7555) (15.4606, -3.7141) (15.5695, -3.6865) knots 0 0 0 0 0.062504 0.093759 0.125013 0.156267 0.187521 0.218774 0.250028 0.281281 0.312533 0.343783 0.359406 0.375028 0.39065 0.406265 0.421876 0.429689 0.437502 0.445312 0.453126 0.460936 0.468749 0.47656 0.484373 0.5 0.515627 0.52344 0.531251 0.539064 0.546874 0.554688 0.562498 0.570311 0.578124 0.593735 0.60935 0.624972 0.640594 0.656217 0.687467 0.718719 0.749972 0.781226 0.812479 0.843733 0.874987 0.906241 0.937496 1 1 1 1 projected
  arc A23 (15.5695, -3.6865) -> (15.7229, -2.9649) centre (0, 0) ccw projected
  spline S15 degree 3 poles (15.7229, -2.9649) (15.6346, -2.8954) (15.5022, -2.7911) (15.3192, -2.6607) (15.1796, -2.5662) (15.0375, -2.4756) (14.8928, -2.3892) (14.7455, -2.3073) (14.5954, -2.2305) (14.4425, -2.1596) (14.2868, -2.095) (14.1538, -2.0496) (14.0467, -2.0157) (13.9687, -1.9835) (13.8945, -1.9433) (13.8259, -1.8939) (13.7761, -1.8442) (13.7408, -1.8003) (13.7193, -1.7641) (13.6988, -1.7271) (13.6848, -1.6873) (13.6722, -1.647) (13.6667, -1.6052) (13.6627, -1.5632) (13.6666, -1.507) (13.6752, -1.4373) (13.6812, -1.3674) (13.6891, -1.3116) (13.7017, -1.2714) (13.7159, -1.2316) (13.7366, -1.1948) (13.7586, -1.1587) (13.7862, -1.1269) (13.8149, -1.0959) (13.8584, -1.0603) (13.9176, -1.022) (13.9949, -0.988) (14.0759, -0.9641) (14.1589, -0.9489) (14.2707, -0.9379) (14.4102, -0.9212) (14.5759, -0.8904) (14.7402, -0.8528) (14.903, -0.8089) (15.0641, -0.7594) (15.2236, -0.705) (15.3815, -0.6459) (15.5376, -0.5825) (15.7438, -0.493) (15.895, -0.4185) (15.9957, -0.3688) knots 0 0 0 0 0.062504 0.093759 0.125013 0.156267 0.187521 0.218774 0.250028 0.281281 0.312533 0.343783 0.359406 0.375028 0.39065 0.406265 0.421876 0.429689 0.437502 0.445312 0.453126 0.460936 0.468749 0.47656 0.484373 0.5 0.515627 0.52344 0.531251 0.539064 0.546874 0.554688 0.562498 0.570311 0.578124 0.593735 0.60935 0.624972 0.640594 0.656217 0.687467 0.718719 0.749972 0.781226 0.812479 0.843733 0.874987 0.906241 0.937496 1 1 1 1 projected
  arc A24 (15.9957, -0.3688) -> (15.9957, 0.3688) centre (0, 0) ccw projected
  spline S16 degree 3 poles (15.9957, 0.3688) (15.895, 0.4185) (15.7438, 0.493) (15.5376, 0.5825) (15.3815, 0.6459) (15.2236, 0.705) (15.0641, 0.7594) (14.903, 0.8089) (14.7402, 0.8528) (14.5759, 0.8904) (14.4102, 0.9212) (14.2707, 0.9379) (14.1589, 0.9489) (14.0759, 0.9641) (13.9949, 0.988) (13.9176, 1.022) (13.8584, 1.0603) (13.8149, 1.0959) (13.7862, 1.1269) (13.7586, 1.1587) (13.7366, 1.1948) (13.7159, 1.2316) (13.7017, 1.2714) (13.6891, 1.3116) (13.6812, 1.3674) (13.6752, 1.4373) (13.6666, 1.507) (13.6627, 1.5632) (13.6667, 1.6052) (13.6722, 1.647) (13.6848, 1.6873) (13.6988, 1.7271) (13.7193, 1.7641) (13.7408, 1.8003) (13.7761, 1.8442) (13.8259, 1.8939) (13.8945, 1.9433) (13.9687, 1.9835) (14.0467, 2.0157) (14.1538, 2.0496) (14.2868, 2.095) (14.4425, 2.1596) (14.5954, 2.2305) (14.7455, 2.3073) (14.8928, 2.3892) (15.0375, 2.4756) (15.1796, 2.5662) (15.3192, 2.6607) (15.5022, 2.7911) (15.6346, 2.8954) (15.7229, 2.9649) knots 0 0 0 0 0.062504 0.093759 0.125013 0.156267 0.187521 0.218774 0.250028 0.281281 0.312533 0.343783 0.359406 0.375028 0.39065 0.406265 0.421876 0.429689 0.437502 0.445312 0.453126 0.460936 0.468749 0.47656 0.484373 0.5 0.515627 0.52344 0.531251 0.539064 0.546874 0.554688 0.562498 0.570311 0.578124 0.593735 0.60935 0.624972 0.640594 0.656217 0.687467 0.718719 0.749972 0.781226 0.812479 0.843733 0.874987 0.906241 0.937496 1 1 1 1 projected
  arc A25 (15.7229, 2.9649) -> (15.5695, 3.6865) centre (0, 0) ccw projected
  arc A26 (14.7629, 6.1691) -> (14.4628, 6.843) centre (0, 0) ccw projected
  arc A27 (13.1576, 9.1037) -> (12.724, 9.7005) centre (0, 0) ccw projected
  arc A28 (10.9773, 11.6404) -> (10.4291, 12.134) centre (0, 0) ccw projected
  arc A29 (8.3173, 13.6683) -> (7.6784, 14.0371) centre (0, 0) ccw projected
  arc A30 (5.2937, 15.0989) -> (4.5922, 15.3268) centre (0, 0) ccw projected
  arc A31 (2.0388, 15.8696) -> (1.3052, 15.9467) centre (0, 0) ccw projected
  arc A32 (-1.3052, 15.9467) -> (-2.0388, 15.8696) centre (0, 0) ccw projected
  arc A33 (-13.6881, 1.3221) -> (-9.3989, -4.5609) centre (-8.7739, 0.3999) ccw
  line L4 (-9.3989, -4.5609) -> (-0.7125, -5.6553)
  arc A34 (-0.7125, -5.6553) -> (0.7125, -5.6553) centre (0, 0) ccw
  line L5 (0.7125, -5.6553) -> (9.3989, -4.5609)
  arc A35 (9.3989, -4.5609) -> (13.6881, 1.3221) centre (8.7739, 0.3999) ccw
  line L6 (11.6778, -2.7619) -> (0.525, -4.1671) projected
  arc A36 (-0.525, -4.1671) -> (0.525, -4.1671) centre (0, 0) ccw projected
  dimension "d27" = 1.5
  dimension "d28" = 5
  constraints: 6 point on circle, 4 end point, 4 tangent, 3 centre point, 2 horizontal alignment, 2 parallel, 1 coincident, 1 equal length, 32 other
  measures "d27" distance between parallel lines of L4 L2
  measures "d28" radius of A35
extrude "Extrusion5" cut sketch "Sketch6" against normal through all contours A33 L4 A34 L5 A35 S16 A24 S15 A23 S14 A22 S13 A21 S12 A20 S11 A19 S10 A18 S9 A17 S8 A16 S7 A15 S6 A14 S5 A13 S4 A12 S3 A11 S2 A10 S1 A9 S0
equation "\"d19\" = 0.5 * d18"
equation "\"Module\" = 1"
equation "\"PressureAngle\" = 20deg"
equation "\"UnitProfileClearance\" = 0.25"
equation "\"UnitRoundRadius\" = 0.35"
equation "\"HeadDiameter\" = 32"
equation "\"RootDiameter\" = 27.5"
equation "\"BaseDiameter\" = 28.19078"
equation "\"FaceWidth\" = 5"
equation "\"HelixAngle\" = 0"
equation "\"UnitCorrection\" = 0"
equation "\"UnitAddendumModification\" = 0"
equation "\"CircularPitch\" = 3.141593"
equation "\"UnitBacklashShift\" = 0"
equation "\"TotalToolShift\" = 0"
equation "\"IsInternal\" = 0"
body "Solid1"
